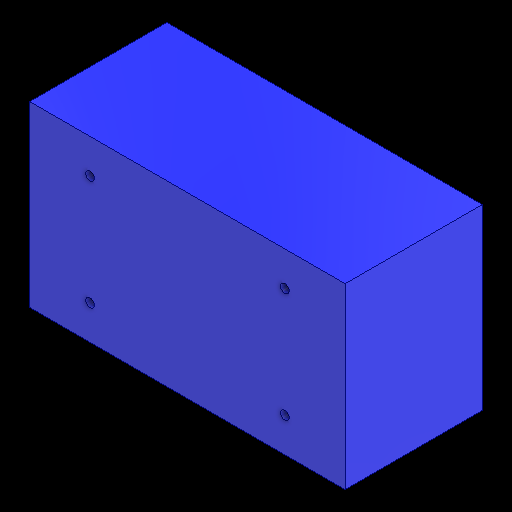
# Autodesk Inventor part: magnet_holder
Saved by Autodesk Inventor 2026.1 (Build 301233000, 233)
## iProperties
Created: 2025-09-30
Part Number: magnet_holder
Material: PC/ABS Plastic
Document SubType Name: Modeling
Designer: drago
Density: 1.1 g/cm^3
Appearance: Blue - Wall Paint - Glossy
Mass: 119.67 g
Surface Area: 407.663 cm^2
Volume: 108.791 cm^3
Author: drago
Autodesk Inventor part; units mm, degrees
ref_plane "YZ Plane" through (0, 0, 0) normal (1, 0, 0) x (0, 1, 0)
ref_plane "XZ Plane" through (0, 0, 0) normal (0, 1, 0) x (-1, 0, 0)
ref_plane "XY Plane" through (0, 0, 0) normal (0, 0, 1) x (1, 0, 0)
sketch "Sketch1" plane through (0, 0, 0) normal (0, 0, 1) x (1, 0, 0)
  line L0 (57.5, -32.5) -> (-57.5, -32.5)
  line L1 (-57.5, -32.5) -> (-57.5, 32.5)
  line L2 (-57.5, 32.5) -> (57.5, 32.5)
  line L3 (57.5, 32.5) -> (57.5, -32.5)
  line L4 (50, -25) -> (-50, -25)
  line L5 (-50, -25) -> (-50, 25)
  line L6 (-50, 25) -> (50, 25)
  line L7 (50, 25) -> (50, -25)
  line L8 (57.5, 0) -> (-57.5, 0) construction
  line L9 (0, -32.5) -> (0, 32.5) construction
  line L10 (-37.5, 32.5) -> (-37.5, 25)
  line L11 (-57.5, 17.5) -> (-50, 17.5)
  line L12 (37.5, -25) -> (37.5, -32.5)
  line L13 (50, -17.5) -> (57.5, -17.5)
  line L14 (-37.5, -25) -> (-37.5, -32.5)
  line L15 (-57.5, -17.5) -> (-50, -17.5)
  line L16 (37.5, 32.5) -> (37.5, 25)
  line L17 (50, 17.5) -> (57.5, 17.5)
  line L18 (-53.75, 28.75) -> (53.75, 28.75) construction
  line L19 (53.75, 28.75) -> (53.75, -28.75) construction
  line L20 (53.75, -28.75) -> (-53.75, -28.75) construction
  line L21 (-53.75, -28.75) -> (-53.75, 28.75) construction
  line L22 (-53.75, 28.75) -> (53.75, -28.75) construction
  line L23 (53.75, 28.75) -> (-53.75, -28.75) construction
  point P0 (0, 0)
  point P1 (-35.5, 20)
  point P2 (35.5, 20)
  point P3 (35.5, -20)
  point P4 (-35.5, -20)
  dimension "d0" = 115
  dimension "d1" = 65
  dimension "d2" = 100
  dimension "d3" = 50
  dimension "d4" = 15
  dimension "d5" = 20
  dimension "d6" = 40
  dimension "d7" = 71
  constraints: 48 end point, 16 point on line, 12 perpendicular, 6 midpoint, 6 parallel, 4 coincident, 4 collinear, 3 horizontal, 3 symmetric about line, 7 other
  measures "d0" distance of L1.end L2.end
  measures "d1" distance between parallel lines of L0 L2
  measures "d2" distance of L5.end L6.end
  measures "d3" distance of L4.end L5.end
  measures "d4" distance between parallel lines of L0 L13
  measures "d5" distance between parallel lines of L3 L12
  measures "d6" distance of point (35.5, 20) point (35.5, -20)
  measures "d7" distance of point (35.5, -20) point (-35.5, -20)
extrude "Extrusion1" add sketch "Sketch1" against normal blind 40 contours L0 L12 L4 L7 L13 L3 | L0 L1 L15 L5 L4 L14 | L17 L7 L6 L16 L2 L3 | L1 L2 L10 L6 L5 L11
extrude "Extrusion2" add sketch "Sketch1" along normal blind 10
hole "Hole1" at (-35.5, 20, 0) at (35.5, 20, 0) at (35.5, -20, 0) at (-35.5, -20, 0) direction (0, 0, 1) diameter 3.2 end through all counterbore diameter 6 counterbore depth 5
extrude "Extrusion8" add sketch "Sketch1" against normal blind 40 contours L0 L14 L4 L12 | L13 L7 L17 L3 | L1 L11 L5 L15 | L16 L6 L10 L2
equation "\"epsilon\" = 0"
body "Solid2"
